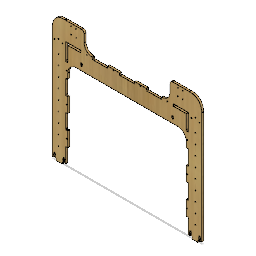
XZ1-plate-IIIS-rev1_8mm v1 (Autodesk Fusion 360 design; units mm, degrees)
Autodesk Fusion 360 part; units mm, degrees
sketch "Basic shape" plane through (0, 0, 0) normal (0, 0, 1) x (1, 0, 0)
  line L0 (-300, 500) -> (300, 500)
  line L1 (300, 500) -> (300, 0)
  line L2 (300, 0) -> (-300, 0)
  line L3 (-300, 0) -> (-300, 500)
  line L4 (-238, 0) -> (238, 0)
  line L5 (238, 0) -> (238, 355)
  line L6 (238, 355) -> (-238, 355)
  line L7 (-238, 355) -> (-238, 0)
  line L8 (300, 500) -> (247, 500)
  line L9 (247, 500) -> (247, 425)
  line L10 (247, 425) -> (300, 425)
  line L11 (300, 425) -> (300, 500)
  line L12 (-300, 500) -> (-247, 500)
  line L13 (-247, 500) -> (-247, 425)
  line L14 (-247, 425) -> (-300, 425)
  line L15 (-300, 425) -> (-300, 500)
  line L16 (247, 425) -> (172, 425)
  line L17 (172, 425) -> (172, 500)
  line L18 (172, 500) -> (247, 500)
  line L19 (247, 500) -> (247, 425)
  line L20 (-247, 425) -> (-172, 425)
  line L21 (-172, 425) -> (-172, 500)
  line L22 (-172, 500) -> (-247, 500)
  line L23 (-247, 500) -> (-247, 425)
  line L24 (-172, 500) -> (172, 500)
  line L25 (172, 500) -> (172, 425)
  line L26 (172, 425) -> (-172, 425)
  line L27 (-172, 425) -> (-172, 500)
  line L28 (-285.5, 0) -> (-260.5, 0)
  line L29 (-260.5, 0) -> (-260.5, -8)
  line L30 (-260.5, -8) -> (-285.5, -8)
  line L31 (-285.5, -8) -> (-285.5, 0)
  line L32 (260.5, 0) -> (285.5, 0)
  line L33 (285.5, 0) -> (285.5, -8)
  line L34 (285.5, -8) -> (260.5, -8)
  line L35 (260.5, -8) -> (260.5, 0)
  dimension "d1" = 500
  dimension "d2" = 600
  dimension "d3" = 53
  dimension "d4" = 53
  dimension "d6" = 62
  dimension "d7" = 75
  dimension "d8" = 75
  dimension "d9" = 75
  dimension "d11" = 25
  dimension "d12" = 8
  dimension "d14" = 14.5
  dimension "d15" = 14.5
  dimension "d16" = 8
  dimension "d17" = 25
  dimension "d102" = 70
  dimension "d111" = 18.5
  dimension "d112" = 23.5
  measures "d1" distance of origin
  measures "d3" distance of L1 L9
  measures "d4" distance of L13 L15
  measures "d6" distance of L1 L5
  measures "d7" distance of L21 L23
  measures "d8" distance of L17 L19
  measures "d9" distance of L24 L26
  measures "d12" distance of origin
  measures "d14" distance of origin L31
  measures "d15" distance of origin L33
  measures "d16" distance of origin
  measures "d102" distance of L6 L26
  measures "d111" distance of origin
extrude "Extrude1" add sketch "Basic shape" along normal blind 8 contours L0 L3 L12 L13 L14 L15 L23 | L0 L13 L20 L21 L22 L23 L27 | L1 L2 L3 L5 L6 L7 L10 L14 L16 L20 L26 L28 L32 | L0 L9 L16 L17 L18 L19 L25 | L2 L28 L29 L30 L31 | L0 L1 L8 L9 L10 L11 L19 | L2 L32 L33 L34 L35
fillet "Fillet1" radius 35 2 edges at (-238, 355, 4) (238, 355, 4)
fillet "Fillet2" radius 32.5 2 edges at (172, 425, 4) (-172, 425, 4)
fillet "Fillet3" radius 10 2 edges at (-172, 500, 4) (172, 500, 4)
sketch "Square+X projected" plane through (0, 0, 8) normal (0, 0, 1) x (1, 0, 0)
  line L0 (300, 500) -> (182, 500)
  arc A0 (182, 500) -> (172, 490) centre (182, 490) ccw
  line L1 (172, 490) -> (172, 457.5)
  arc A1 (139.5, 425) -> (172, 457.5) centre (139.5, 457.5) ccw
  line L2 (139.5, 425) -> (-139.5, 425)
  arc A2 (-172, 457.5) -> (-139.5, 425) centre (-139.5, 457.5) ccw
  line L3 (-172, 457.5) -> (-172, 490)
  arc A3 (-172, 490) -> (-182, 500) centre (-182, 490) ccw
  line L4 (-182, 500) -> (-247, 500)
  line L5 (-300, 0) -> (-285.5, 0)
  line L6 (-285.5, 0) -> (-285.5, -8)
  line L7 (-285.5, -8) -> (-260.5, -8)
  line L8 (-260.5, -8) -> (-260.5, 0)
  line L9 (-260.5, 0) -> (-238, 0)
  line L10 (-238, 0) -> (-238, 320)
  arc A4 (-203, 355) -> (-238, 320) centre (-203, 320) ccw
  line L11 (-203, 355) -> (203, 355)
  arc A5 (238, 320) -> (203, 355) centre (203, 320) ccw
  line L12 (238, 320) -> (238, 0)
  line L13 (238, 0) -> (260.5, 0)
  line L14 (260.5, 0) -> (260.5, -8)
  line L15 (260.5, -8) -> (285.5, -8)
  line L16 (285.5, -8) -> (285.5, 0)
  line L17 (285.5, 0) -> (300, 0)
  line L18 (300, 0) -> (300, 500)
  line L19 (-238, 0) -> (-246, 0) construction
  line L20 (-246, 0) -> (-246, 500) construction
  line L21 (-246, 500) -> (-238, 500) construction
  line L22 (-238, 500) -> (-238, 0) construction
  line L23 (-300, 425) -> (300, 425) construction
  line L24 (300, 425) -> (300, 417) construction
  line L25 (300, 417) -> (-300, 417) construction
  line L26 (-300, 417) -> (-300, 425) construction
  line L27 (-247, 500) -> (-300, 500)
  dimension "d27" = 8
  dimension "d34" = 8
  dimension "d107" = 75
sketch "Square+X joints" plane through (0, 0, 0) normal (0, 0, 1) x (1, 0, 0)
  line L0 (-238, 0) -> (-246, 0)
  line L1 (-246, 0) -> (-246, 60)
  line L2 (-246, 60) -> (-238, 60)
  line L3 (-238, 60) -> (-238, 0)
  line L4 (-246, 0) -> (-246, 500)
  line L5 (-238, 119) -> (-246, 119)
  line L6 (-246, 119) -> (-246, 179)
  line L7 (-246, 179) -> (-238, 179)
  line L8 (-238, 179) -> (-238, 119)
  line L9 (-238, 320) -> (-238, 0)
  line L10 (-238, 238) -> (-246, 238)
  line L11 (-246, 238) -> (-246, 298)
  line L12 (-246, 298) -> (-238, 298)
  line L13 (-238, 298) -> (-238, 238)
  line L14 (-246, 238) -> (-246, 179) construction
  line L15 (-246, 119) -> (-246, 60) construction
  line L16 (-238, 357) -> (-246, 357)
  line L17 (-246, 357) -> (-246, 417)
  line L18 (-246, 417) -> (-238, 417)
  line L19 (-238, 417) -> (-238, 357)
  line L20 (-246, 357) -> (-246, 298) construction
  line L21 (30, 425) -> (-30, 425)
  line L22 (-30, 425) -> (-30, 417)
  line L23 (-30, 417) -> (30, 417)
  line L24 (30, 417) -> (30, 425)
  line L25 (300, 417) -> (-300, 417)
  line L26 (-78, 425) -> (-138, 425)
  line L27 (-138, 425) -> (-138, 417)
  line L28 (-138, 417) -> (-78, 417)
  line L29 (-78, 417) -> (-78, 425)
  line L30 (-300, 425) -> (300, 425)
  line L31 (-186, 425) -> (-246, 425)
  line L32 (-30, 417) -> (-78, 417) construction
  line L33 (78, 425) -> (138, 425)
  line L34 (138, 425) -> (138, 417)
  line L35 (138, 417) -> (78, 417)
  line L36 (78, 417) -> (78, 425)
  line L37 (186, 425) -> (246, 425)
  line L38 (246, 425) -> (246, 417)
  line L39 (246, 417) -> (186, 417)
  line L40 (186, 417) -> (186, 425)
  line L41 (186, 417) -> (138, 417) construction
  line L42 (78, 417) -> (30, 417) construction
  line L43 (300, 417) -> (246, 417) construction
  line L44 (-138, 417) -> (-186, 417) construction
  line L45 (-186, 425) -> (-186, 417)
  line L46 (-246, 417) -> (-246, 425)
  line L47 (-246, 417) -> (-186, 417)
  line L48 (-246, 417) -> (-300, 417) construction
  dimension "d28" = 60
  dimension "d29" = 60
  dimension "d30" = 60
  dimension "d31" = 60
  dimension "d33" = 58.3333
  dimension "d35" = 60
  dimension "d36" = 60
  dimension "d37" = 60
  dimension "d44" = 31.6667
  dimension "d46" = 60
  dimension "d47" = 60
extrude "Extrude2" cut sketch "Square+X joints" along normal blind 8 contours L0 L1 L2 L3 L4 L9 | L4 L5 L6 L7 L8 L9 | L4 L9 L10 L11 L12 L13
extrude "Extrude3" cut sketch "Square+X joints" along normal through all contours L4 L16 L17 L18 L19 L25 L47 | L4 L18 L25 L30 L31 L45 L46 L47 | L25 L26 L27 L28 L29 L30 | L21 L22 L23 L24 L25 L30
mirror "Mirror1" about plane through (0, 0, 0) normal (1, 0, 0) of "Extrude2", "Extrude3"
sketch "Square+X joints holes" plane through (0, 0, 8) normal (0, 0, 1) x (1, 0, 0)
  line L0 (246, 60) -> (246, 0)
  line L1 (246, 0) -> (260.5, 0)
  line L2 (260.5, 0) -> (260.5, -8)
  line L3 (260.5, -8) -> (285.5, -8)
  line L4 (285.5, -8) -> (285.5, 0)
  line L5 (285.5, 0) -> (300, 0)
  line L6 (300, 0) -> (300, 500)
  line L7 (300, 500) -> (182, 500)
  arc A0 (182, 500) -> (172, 490) centre (182, 490) ccw
  line L8 (172, 490) -> (172, 457.5)
  arc A1 (139.5, 425) -> (172, 457.5) centre (139.5, 457.5) ccw
  line L9 (78, 425) -> (30, 425)
  arc A2 (-172, 457.5) -> (-139.5, 425) centre (-139.5, 457.5) ccw
  line L10 (-172, 457.5) -> (-172, 490)
  arc A3 (-172, 490) -> (-182, 500) centre (-182, 490) ccw
  line L11 (-182, 500) -> (-247, 500)
  line L12 (-300, 500) -> (-300, 0)
  line L13 (-300, 0) -> (-285.5, 0)
  line L14 (-285.5, 0) -> (-285.5, -8)
  line L15 (-285.5, -8) -> (-260.5, -8)
  line L16 (-260.5, -8) -> (-260.5, 0)
  line L17 (-260.5, 0) -> (-246, 0)
  line L18 (-246, 0) -> (-246, 60)
  line L19 (-246, 60) -> (-238, 60)
  line L20 (-238, 60) -> (-238, 119)
  line L21 (-238, 119) -> (-246, 119)
  line L22 (-246, 119) -> (-246, 179)
  line L23 (-246, 179) -> (-238, 179)
  line L24 (-238, 179) -> (-238, 238)
  line L25 (-238, 238) -> (-246, 238)
  line L26 (-246, 238) -> (-246, 298)
  line L27 (-246, 298) -> (-238, 298)
  arc A4 (-203, 355) -> (-238, 320) centre (-203, 320) ccw
  line L28 (-203, 355) -> (203, 355)
  arc A5 (238, 320) -> (203, 355) centre (203, 320) ccw
  line L29 (238, 298) -> (246, 298)
  line L30 (246, 298) -> (246, 238)
  line L31 (246, 238) -> (238, 238)
  line L32 (238, 320) -> (238, 298)
  line L33 (238, 179) -> (246, 179)
  line L34 (246, 179) -> (246, 119)
  line L35 (246, 119) -> (238, 119)
  line L36 (238, 119) -> (238, 60)
  line L37 (238, 60) -> (246, 60)
  circle A6 centre (-242, 89.5) radius 2
  circle A7 centre (-242, 208.5) radius 2
  circle A8 centre (-242, 327.338) radius 2
  circle A9 centre (-54, 421) radius 2
  circle A10 centre (-162, 421) radius 2
  line L38 (-30, 425) -> (-30, 417)
  circle A11 centre (-275, 421) radius 2
  line L39 (-30, 425) -> (-78, 425)
  line L40 (-246, 425) -> (-300, 500) construction
  line L41 (-138, 425) -> (-138, 417)
  line L42 (-138, 425) -> (-186, 425) construction
  line L43 (-247, 500) -> (-300, 500)
  line L44 (-238, 298) -> (-238, 320)
  line L45 (78, 417) -> (78, 425)
  line L46 (30, 425) -> (30, 417)
  line L47 (30, 417) -> (-30, 417)
  line L48 (-30, 417) -> (-30, 425)
  line L49 (-30, 425) -> (-78, 425)
  line L50 (-78, 425) -> (-78, 417)
  line L51 (-78, 417) -> (-138, 417)
  line L52 (-138, 417) -> (-138, 425)
  line L53 (-138, 425) -> (-139.5, 425)
  line L54 (238, 238) -> (238, 179)
  line L55 (139.5, 425) -> (138, 425)
  line L56 (138, 425) -> (138, 417)
  line L57 (138, 417) -> (78, 417)
  line L58 (238, 417) -> (186, 417)
  line L59 (186, 417) -> (186, 425)
  line L60 (186, 425) -> (246, 425)
  line L61 (246, 425) -> (246, 357)
  line L62 (246, 357) -> (238, 357)
  line L63 (238, 357) -> (238, 417)
  line L64 (-238, 357) -> (-246, 357)
  line L65 (-246, 357) -> (-246, 425)
  line L66 (-246, 425) -> (-186, 425)
  line L67 (-186, 425) -> (-186, 417)
  line L68 (-186, 417) -> (-238, 417)
  line L69 (-238, 417) -> (-238, 357)
  dimension "d49" = 29.1667
  dimension "d50" = 29.338
  dimension "d51" = 4
  dimension "d52" = 4
  dimension "d53" = 4
  dimension "d59" = 4
  dimension "d60" = 4
  dimension "d61" = 4
  dimension "d101" = 275
  measures "d51" diameter of A6
  measures "d52" diameter of A7
  measures "d53" diameter of A8
  measures "d59" diameter of A11
  measures "d60" diameter of A10
  measures "d61" diameter of A9
  measures "d101" distance of origin
extrude "Extrude4" cut sketch "Square+X joints holes" against normal through all contours A6 | A7 | A8 | A9 | A10 | A11
mirror "Mirror2" about plane through (0, 0, 0) normal (1, 0, 0) of "Extrude4"
sketch "Linear rail" plane through (0, 0, 8) normal (0, 0, 1) x (1, 0, 0)
  circle A0 centre (242, 89.5) radius 2
  circle A1 centre (162, 421) radius 2
  circle A2 centre (242, 208.5) radius 2
  circle A3 centre (275, 421) radius 2
  circle A4 centre (-54, 421) radius 2
  circle A5 centre (-242, 89.5) radius 2
  circle A6 centre (-162, 421) radius 2
  circle A7 centre (-242, 208.5) radius 2
  circle A8 centre (-275, 421) radius 2
  line L0 (246, 60) -> (246, 0)
  line L1 (246, 0) -> (260.5, 0)
  line L2 (260.5, 0) -> (260.5, -8)
  line L3 (260.5, -8) -> (285.5, -8)
  line L4 (285.5, -8) -> (285.5, 0)
  line L5 (285.5, 0) -> (300, 0)
  line L6 (300, 0) -> (300, 500)
  line L7 (300, 500) -> (182, 500)
  arc A9 (182, 500) -> (172, 490) centre (182, 490) ccw
  line L8 (172, 490) -> (172, 457.5)
  arc A10 (139.5, 425) -> (172, 457.5) centre (139.5, 457.5) ccw
  line L9 (78, 425) -> (30, 425)
  arc A11 (-172, 457.5) -> (-139.5, 425) centre (-139.5, 457.5) ccw
  line L10 (-172, 457.5) -> (-172, 490)
  arc A12 (-172, 490) -> (-182, 500) centre (-182, 490) ccw
  line L11 (-182, 500) -> (-247, 500)
  line L12 (-300, 500) -> (-300, 0)
  line L13 (-300, 0) -> (-285.5, 0)
  line L14 (-285.5, 0) -> (-285.5, -8)
  line L15 (-285.5, -8) -> (-260.5, -8)
  line L16 (-260.5, -8) -> (-260.5, 0)
  line L17 (-260.5, 0) -> (-246, 0)
  line L18 (-246, 0) -> (-246, 60)
  line L19 (-246, 60) -> (-238, 60)
  line L20 (-238, 60) -> (-238, 119)
  line L21 (-238, 119) -> (-246, 119)
  line L22 (-246, 119) -> (-246, 179)
  line L23 (-246, 179) -> (-238, 179)
  line L24 (-238, 179) -> (-238, 238)
  line L25 (-238, 238) -> (-246, 238)
  line L26 (-246, 238) -> (-246, 298)
  line L27 (-246, 298) -> (-238, 298)
  arc A13 (-203, 355) -> (-238, 320) centre (-203, 320) ccw
  line L28 (-203, 355) -> (203, 355)
  arc A14 (238, 320) -> (203, 355) centre (203, 320) ccw
  line L29 (238, 298) -> (246, 298)
  line L30 (246, 298) -> (246, 238)
  line L31 (246, 238) -> (238, 238)
  line L32 (238, 320) -> (238, 298)
  line L33 (238, 179) -> (246, 179)
  line L34 (246, 179) -> (246, 119)
  line L35 (246, 119) -> (238, 119)
  line L36 (238, 119) -> (238, 60)
  line L37 (238, 60) -> (246, 60)
  circle A15 centre (-275, 368.1667) radius 1.5
  line L38 (-247, 500) -> (-300, 500)
  circle A16 centre (54, 421) radius 2
  circle A17 centre (242, 327.338) radius 2
  circle A18 centre (-242, 327.338) radius 2
  line L39 (-238, 298) -> (-238, 320)
  line L40 (78, 417) -> (78, 425)
  line L41 (30, 425) -> (30, 417)
  line L42 (30, 417) -> (-30, 417)
  line L43 (-30, 417) -> (-30, 425)
  line L44 (-30, 425) -> (-78, 425)
  line L45 (-78, 425) -> (-78, 417)
  line L46 (-78, 417) -> (-138, 417)
  line L47 (-138, 417) -> (-138, 425)
  line L48 (-138, 425) -> (-139.5, 425)
  line L49 (238, 238) -> (238, 179)
  line L50 (139.5, 425) -> (138, 425)
  line L51 (138, 425) -> (138, 417)
  line L52 (138, 417) -> (78, 417)
  line L53 (238, 417) -> (186, 417)
  line L54 (186, 417) -> (186, 425)
  line L55 (186, 425) -> (246, 425)
  line L56 (246, 425) -> (246, 357)
  line L57 (246, 357) -> (238, 357)
  line L58 (238, 357) -> (238, 417)
  line L59 (-238, 357) -> (-246, 357)
  line L60 (-246, 357) -> (-246, 425)
  line L61 (-246, 425) -> (-186, 425)
  line L62 (-186, 425) -> (-186, 417)
  line L63 (-186, 417) -> (-238, 417)
  line L64 (-238, 417) -> (-238, 357)
  dimension "d63" = 275
  dimension "d64" = 3
  measures "d63" distance of origin
  measures "d64" diameter of A15
extrude "Extrude5" cut sketch "Linear rail" against normal through all contours A15
pattern_linear "R-Pattern1" count 9 spacing 40 along (0, -1, 0) of "Extrude5"
mirror "Mirror3" about plane through (0, 0, 0) normal (1, 0, 0) of "Extrude5", "R-Pattern1"
sketch "Motor fixation" plane through (0, 0, 8) normal (0, 0, 1) x (1, 0, 0)
  circle A0 centre (275, 368.1667) radius 1.5
  circle A1 centre (-275, 48.1667) radius 1.5
  circle A2 centre (-275, 88.1667) radius 1.5
  circle A3 centre (-275, 128.1667) radius 1.5
  circle A4 centre (-275, 168.1667) radius 1.5
  circle A5 centre (-275, 208.1667) radius 1.5
  circle A6 centre (-275, 248.1667) radius 1.5
  circle A7 centre (-275, 288.1667) radius 1.5
  circle A8 centre (-275, 328.1667) radius 1.5
  circle A9 centre (-275, 368.1667) radius 1.5
  circle A10 centre (242, 89.5) radius 2
  circle A11 centre (162, 421) radius 2
  circle A12 centre (242, 208.5) radius 2
  circle A13 centre (275, 421) radius 2
  circle A14 centre (-54, 421) radius 2
  circle A15 centre (-242, 89.5) radius 2
  circle A16 centre (-162, 421) radius 2
  circle A17 centre (-242, 208.5) radius 2
  circle A18 centre (-275, 421) radius 2
  line L0 (246, 60) -> (246, 0)
  line L1 (246, 0) -> (260.5, 0)
  line L2 (260.5, 0) -> (260.5, -8)
  line L3 (260.5, -8) -> (285.5, -8)
  line L4 (285.5, -8) -> (285.5, 0)
  line L5 (285.5, 0) -> (300, 0)
  line L6 (300, 0) -> (300, 500)
  line L7 (300, 500) -> (182, 500)
  arc A19 (182, 500) -> (172, 490) centre (182, 490) ccw
  line L8 (172, 490) -> (172, 457.5)
  arc A20 (139.5, 425) -> (172, 457.5) centre (139.5, 457.5) ccw
  line L9 (78, 425) -> (30, 425)
  arc A21 (-172, 457.5) -> (-139.5, 425) centre (-139.5, 457.5) ccw
  line L10 (-172, 457.5) -> (-172, 490)
  arc A22 (-172, 490) -> (-182, 500) centre (-182, 490) ccw
  line L11 (-182, 500) -> (-247, 500)
  line L12 (-300, 500) -> (-300, 0)
  line L13 (-300, 0) -> (-285.5, 0)
  line L14 (-285.5, 0) -> (-285.5, -8)
  line L15 (-285.5, -8) -> (-260.5, -8)
  line L16 (-260.5, -8) -> (-260.5, 0)
  line L17 (-260.5, 0) -> (-246, 0)
  line L18 (-246, 0) -> (-246, 60)
  line L19 (-246, 60) -> (-238, 60)
  line L20 (-238, 60) -> (-238, 119)
  line L21 (-238, 119) -> (-246, 119)
  line L22 (-246, 119) -> (-246, 179)
  line L23 (-246, 179) -> (-238, 179)
  line L24 (-238, 179) -> (-238, 238)
  line L25 (-238, 238) -> (-246, 238)
  line L26 (-246, 238) -> (-246, 298)
  line L27 (-246, 298) -> (-238, 298)
  arc A23 (-203, 355) -> (-238, 320) centre (-203, 320) ccw
  line L28 (-203, 355) -> (203, 355)
  arc A24 (238, 320) -> (203, 355) centre (203, 320) ccw
  line L29 (238, 298) -> (246, 298)
  line L30 (246, 298) -> (246, 238)
  line L31 (246, 238) -> (238, 238)
  line L32 (238, 320) -> (238, 298)
  line L33 (238, 179) -> (246, 179)
  line L34 (246, 179) -> (246, 119)
  line L35 (246, 119) -> (238, 119)
  line L36 (238, 119) -> (238, 60)
  line L37 (238, 60) -> (246, 60)
  line L38 (-229.5, 487.99) -> (-199.5, 487.99)
  arc A25 (-199.5, 487.99) -> (-199.5, 492.01) centre (-199.5, 490) ccw
  line L39 (-199.5, 492.01) -> (-229.5, 492.01)
  arc A26 (-229.5, 492.01) -> (-229.5, 487.99) centre (-229.5, 490) ccw
  line L40 (-229.5, 490) -> (-199.5, 490) construction
  line L41 (-229.5, 457.99) -> (-199.5, 457.99)
  arc A27 (-199.5, 457.99) -> (-199.5, 462.01) centre (-199.5, 460) ccw
  line L42 (-199.5, 462.01) -> (-229.5, 462.01)
  arc A28 (-229.5, 462.01) -> (-229.5, 457.99) centre (-229.5, 460) ccw
  line L43 (-229.5, 460) -> (-199.5, 460) construction
  line L44 (-214.5, 490) -> (-214.5, 460) construction
  circle A29 centre (275, 48.1667) radius 1.5
  circle A30 centre (275, 88.1667) radius 1.5
  circle A31 centre (275, 128.1667) radius 1.5
  circle A32 centre (275, 168.1667) radius 1.5
  circle A33 centre (275, 208.1667) radius 1.5
  circle A34 centre (275, 248.1667) radius 1.5
  circle A35 centre (275, 288.1667) radius 1.5
  circle A36 centre (275, 328.1667) radius 1.5
  line L45 (-247, 500) -> (-300, 500)
  circle A37 centre (54, 421) radius 2
  circle A38 centre (242, 327.338) radius 2
  circle A39 centre (-242, 327.338) radius 2
  line L46 (-238, 298) -> (-238, 320)
  line L47 (78, 417) -> (78, 425)
  line L48 (30, 425) -> (30, 417)
  line L49 (30, 417) -> (-30, 417)
  line L50 (-30, 417) -> (-30, 425)
  line L51 (-30, 425) -> (-78, 425)
  line L52 (-78, 425) -> (-78, 417)
  line L53 (-78, 417) -> (-138, 417)
  line L54 (-138, 417) -> (-138, 425)
  line L55 (-138, 425) -> (-139.5, 425)
  line L56 (238, 238) -> (238, 179)
  line L57 (139.5, 425) -> (138, 425)
  line L58 (138, 425) -> (138, 417)
  line L59 (138, 417) -> (78, 417)
  line L60 (238, 417) -> (186, 417)
  line L61 (186, 417) -> (186, 425)
  line L62 (186, 425) -> (246, 425)
  line L63 (246, 425) -> (246, 357)
  line L64 (246, 357) -> (238, 357)
  line L65 (238, 357) -> (238, 417)
  line L66 (-238, 357) -> (-246, 357)
  line L67 (-246, 357) -> (-246, 425)
  line L68 (-246, 425) -> (-186, 425)
  line L69 (-186, 425) -> (-186, 417)
  line L70 (-186, 417) -> (-238, 417)
  line L71 (-238, 417) -> (-238, 357)
  circle A40 centre (-204.5, 490) radius 2.01
  circle A41 centre (-224.5, 490) radius 2.01
  circle A42 centre (-204.5, 460) radius 2.01
  circle A43 centre (-224.5, 460) radius 2.01
  line L72 (-186, 380) -> (-186, 374)
  arc A44 (-186, 374) -> (-180, 374) centre (-183, 374) ccw
  line L73 (-180, 374) -> (-180, 380)
  arc A45 (-180, 380) -> (-186, 380) centre (-183, 380) ccw
  line L74 (-183, 380) -> (-183, 374) construction
  dimension "d73" = 30
  dimension "d74" = 30
  dimension "d75" = 30
  dimension "d76" = 2.01
  dimension "d77" = 2.01
  dimension "d512" = 10
  dimension "d513" = 20
  dimension "d514" = 10
  dimension "d515" = 20
  dimension "d517" = 10
  dimension "d519" = 183
  dimension "d520" = 380
  dimension "d521" = 6
  dimension "d522" = 3
  measures "d519" distance of origin
  measures "d520" distance of origin
  measures "d522" distance of L73
extrude "Extrude6" cut sketch "Motor fixation" against normal through all contours A41 | A40 | A43 | A42 | L72 A44 L73 A45
mirror "Mirror4" about plane through (0, 0, 0) normal (1, 0, 0) of "Extrude6"
sketch "T slots" plane through (0, 0, 8) normal (0, 0, 1) x (1, 0, 0)
  circle A0 centre (275, 368.1667) radius 1.5
  circle A1 centre (-275, 48.1667) radius 1.5
  circle A2 centre (-275, 88.1667) radius 1.5
  circle A3 centre (-275, 128.1667) radius 1.5
  circle A4 centre (-275, 168.1667) radius 1.5
  circle A5 centre (-275, 208.1667) radius 1.5
  circle A6 centre (-275, 248.1667) radius 1.5
  circle A7 centre (-275, 288.1667) radius 1.5
  circle A8 centre (-275, 328.1667) radius 1.5
  circle A9 centre (-275, 368.1667) radius 1.5
  circle A10 centre (242, 89.5) radius 2
  circle A11 centre (162, 421) radius 2
  circle A12 centre (242, 208.5) radius 2
  circle A13 centre (275, 421) radius 2
  circle A14 centre (-54, 421) radius 2
  circle A15 centre (-242, 89.5) radius 2
  circle A16 centre (-162, 421) radius 2
  circle A17 centre (-242, 208.5) radius 2
  circle A18 centre (-275, 421) radius 2
  line L0 (246, 60) -> (246, 0)
  line L1 (246, 0) -> (260.5, 0)
  line L2 (260.5, 0) -> (260.5, -8)
  line L3 (260.5, -8) -> (285.5, -8)
  line L4 (285.5, -8) -> (285.5, 0)
  line L5 (285.5, 0) -> (300, 0)
  line L6 (300, 0) -> (300, 500)
  line L7 (300, 500) -> (182, 500)
  arc A19 (182, 500) -> (172, 490) centre (182, 490) ccw
  line L8 (172, 490) -> (172, 457.5)
  arc A20 (139.5, 425) -> (172, 457.5) centre (139.5, 457.5) ccw
  line L9 (78, 425) -> (30, 425)
  arc A21 (-172, 457.5) -> (-139.5, 425) centre (-139.5, 457.5) ccw
  line L10 (-172, 457.5) -> (-172, 490)
  arc A22 (-172, 490) -> (-182, 500) centre (-182, 490) ccw
  line L11 (-182, 500) -> (-247, 500)
  line L12 (-300, 500) -> (-300, 0)
  line L13 (-300, 0) -> (-285.5, 0)
  line L14 (-285.5, 0) -> (-285.5, -8)
  line L15 (-285.5, -8) -> (-260.5, -8)
  line L16 (-260.5, -8) -> (-260.5, 0)
  line L17 (-260.5, 0) -> (-246, 0)
  line L18 (-246, 0) -> (-246, 60)
  line L19 (-246, 60) -> (-238, 60)
  line L20 (-238, 60) -> (-238, 119)
  line L21 (-238, 119) -> (-246, 119)
  line L22 (-246, 119) -> (-246, 179)
  line L23 (-246, 179) -> (-238, 179)
  line L24 (-238, 179) -> (-238, 238)
  line L25 (-238, 238) -> (-246, 238)
  line L26 (-246, 238) -> (-246, 298)
  line L27 (-246, 298) -> (-238, 298)
  arc A23 (-203, 355) -> (-238, 320) centre (-203, 320) ccw
  line L28 (-203, 355) -> (203, 355)
  arc A24 (238, 320) -> (203, 355) centre (203, 320) ccw
  line L29 (238, 298) -> (246, 298)
  line L30 (246, 298) -> (246, 238)
  line L31 (246, 238) -> (238, 238)
  line L32 (238, 320) -> (238, 298)
  line L33 (238, 179) -> (246, 179)
  line L34 (246, 179) -> (246, 119)
  line L35 (246, 119) -> (238, 119)
  line L36 (238, 119) -> (238, 60)
  line L37 (238, 60) -> (246, 60)
  line L38 (-293.51, 0) -> (-289.49, 0)
  line L39 (-289.49, 0) -> (-289.49, 17.5)
  line L40 (-289.49, 17.5) -> (-293.51, 17.5)
  line L41 (-293.51, 17.5) -> (-293.51, 0)
  line L42 (-294.98, 12.5) -> (-287.98, 12.5)
  line L43 (-287.98, 12.5) -> (-287.98, 5)
  line L44 (-287.98, 5) -> (-294.98, 5)
  line L45 (-294.98, 5) -> (-294.98, 12.5)
  circle A25 centre (275, 48.1667) radius 1.5
  circle A26 centre (275, 88.1667) radius 1.5
  circle A27 centre (275, 128.1667) radius 1.5
  circle A28 centre (275, 168.1667) radius 1.5
  circle A29 centre (275, 208.1667) radius 1.5
  circle A30 centre (275, 248.1667) radius 1.5
  circle A31 centre (275, 288.1667) radius 1.5
  circle A32 centre (275, 328.1667) radius 1.5
  line L46 (-247, 500) -> (-300, 500)
  circle A33 centre (54, 421) radius 2
  circle A34 centre (242, 327.338) radius 2
  circle A35 centre (-242, 327.338) radius 2
  line L47 (-238, 298) -> (-238, 320)
  line L48 (78, 417) -> (78, 425)
  line L49 (30, 425) -> (30, 417)
  line L50 (30, 417) -> (-30, 417)
  line L51 (-30, 417) -> (-30, 425)
  line L52 (-30, 425) -> (-78, 425)
  line L53 (-78, 425) -> (-78, 417)
  line L54 (-78, 417) -> (-138, 417)
  line L55 (-138, 417) -> (-138, 425)
  line L56 (-138, 425) -> (-139.5, 425)
  line L57 (139.5, 425) -> (138, 425)
  line L58 (138, 425) -> (138, 417)
  line L59 (138, 417) -> (78, 417)
  line L60 (238, 417) -> (186, 417)
  line L61 (186, 417) -> (186, 425)
  line L62 (186, 425) -> (246, 425)
  line L63 (246, 425) -> (246, 357)
  line L64 (246, 357) -> (238, 357)
  line L65 (238, 357) -> (238, 417)
  line L66 (-238, 357) -> (-246, 357)
  line L67 (-246, 357) -> (-246, 425)
  line L68 (-246, 425) -> (-186, 425)
  line L69 (-186, 425) -> (-186, 417)
  line L70 (-186, 417) -> (-238, 417)
  line L71 (-238, 417) -> (-238, 357)
  circle A36 centre (204.5, 490) radius 2.01
  circle A37 centre (224.5, 460) radius 2.01
  circle A38 centre (224.5, 490) radius 2.01
  circle A39 centre (204.5, 460) radius 2.01
  circle A40 centre (-204.5, 490) radius 2.01
  circle A41 centre (-224.5, 460) radius 2.01
  circle A42 centre (-224.5, 490) radius 2.01
  circle A43 centre (-204.5, 460) radius 2.01
  line L72 (186, 380) -> (186, 374)
  arc A44 (180, 374) -> (186, 374) centre (183, 374) ccw
  line L73 (180, 374) -> (180, 380)
  arc A45 (186, 380) -> (180, 380) centre (183, 380) ccw
  line L74 (-180, 380) -> (-180, 374)
  arc A46 (-186, 374) -> (-180, 374) centre (-183, 374) ccw
  line L75 (-186, 374) -> (-186, 380)
  arc A47 (-180, 380) -> (-186, 380) centre (-183, 380) ccw
  line L76 (238, 238) -> (238, 179)
  dimension "d82" = 4.02
  dimension "d84" = 7
  dimension "d85" = 7.5
  dimension "d86" = 5
  dimension "d87" = 17.5
  dimension "d103" = 1.51
  dimension "d511" = 6
  measures "d86" distance of origin L44
  measures "d87" distance of origin
  measures "d103" distance of origin
extrude "Extrude7" cut sketch "T slots" against normal through all contours L13 L38 L39 L41 L44 | L39 L41 L42 L44 | L39 L42 L43 L44 | L41 L42 L44 L45 | L39 L40 L41 L42
pattern_linear "R-Pattern2" count 2 spacing 37 along (1, 0, 0) of "Extrude7"
mirror "Mirror5" about plane through (0, 0, 0) normal (1, 0, 0) of "Extrude7", "R-Pattern2"
sketch "SK8" plane through (0, 0, 8) normal (0, 0, 1) x (1, 0, 0)
  circle A0 centre (275, 48.1667) radius 1.5
  circle A1 centre (275, 88.1667) radius 1.5
  circle A2 centre (275, 128.1667) radius 1.5
  circle A3 centre (275, 168.1667) radius 1.5
  circle A4 centre (275, 208.1667) radius 1.5
  circle A5 centre (275, 248.1667) radius 1.5
  circle A6 centre (275, 288.1667) radius 1.5
  circle A7 centre (275, 328.1667) radius 1.5
  circle A8 centre (275, 368.1667) radius 1.5
  circle A9 centre (-275, 48.1667) radius 1.5
  circle A10 centre (-275, 88.1667) radius 1.5
  circle A11 centre (-275, 128.1667) radius 1.5
  circle A12 centre (-275, 168.1667) radius 1.5
  circle A13 centre (-275, 208.1667) radius 1.5
  circle A14 centre (-275, 248.1667) radius 1.5
  circle A15 centre (-275, 288.1667) radius 1.5
  circle A16 centre (-275, 328.1667) radius 1.5
  circle A17 centre (-275, 368.1667) radius 1.5
  circle A18 centre (242, 89.5) radius 2
  circle A19 centre (162, 421) radius 2
  circle A20 centre (242, 208.5) radius 2
  circle A21 centre (275, 421) radius 2
  circle A22 centre (-54, 421) radius 2
  circle A23 centre (-242, 89.5) radius 2
  circle A24 centre (-162, 421) radius 2
  circle A25 centre (-242, 208.5) radius 2
  circle A26 centre (-275, 421) radius 2
  line L0 (252.49, 0) -> (252.49, 5)
  line L1 (252.49, 5) -> (250.98, 5)
  line L2 (250.98, 5) -> (250.98, 12.5)
  line L3 (250.98, 12.5) -> (252.49, 12.5)
  line L4 (252.49, 12.5) -> (252.49, 17.5)
  line L5 (252.49, 17.5) -> (256.51, 17.5)
  line L6 (256.51, 17.5) -> (256.51, 12.5)
  line L7 (256.51, 12.5) -> (257.98, 12.5)
  line L8 (257.98, 12.5) -> (257.98, 5)
  line L9 (257.98, 5) -> (256.51, 5)
  line L10 (256.51, 5) -> (256.51, 0)
  line L11 (260.5, 0) -> (260.5, -8)
  line L12 (260.5, -8) -> (285.5, -8)
  line L13 (285.5, -8) -> (285.5, 0)
  line L14 (285.5, 0) -> (289.49, 0)
  line L15 (289.49, 0) -> (289.49, 5)
  line L16 (289.49, 5) -> (287.98, 5)
  line L17 (287.98, 5) -> (287.98, 12.5)
  line L18 (287.98, 12.5) -> (289.49, 12.5)
  line L19 (289.49, 12.5) -> (289.49, 17.5)
  line L20 (289.49, 17.5) -> (293.51, 17.5)
  line L21 (293.51, 17.5) -> (293.51, 12.5)
  line L22 (293.51, 12.5) -> (294.98, 12.5)
  line L23 (294.98, 12.5) -> (294.98, 5)
  line L24 (294.98, 5) -> (293.51, 5)
  line L25 (293.51, 5) -> (293.51, 0)
  line L26 (293.51, 0) -> (300, 0)
  line L27 (300, 0) -> (300, 500)
  line L28 (300, 500) -> (182, 500)
  arc A27 (182, 500) -> (172, 490) centre (182, 490) ccw
  line L29 (172, 490) -> (172, 457.5)
  arc A28 (139.5, 425) -> (172, 457.5) centre (139.5, 457.5) ccw
  line L30 (139.5, 425) -> (138, 425)
  arc A29 (-172, 457.5) -> (-139.5, 425) centre (-139.5, 457.5) ccw
  line L31 (-172, 457.5) -> (-172, 490)
  arc A30 (-172, 490) -> (-182, 500) centre (-182, 490) ccw
  line L32 (-182, 500) -> (-247, 500)
  line L33 (-300, 500) -> (-300, 0)
  line L34 (-300, 0) -> (-293.51, 0)
  line L35 (-293.51, 0) -> (-293.51, 5)
  line L36 (-293.51, 5) -> (-294.98, 5)
  line L37 (-294.98, 5) -> (-294.98, 12.5)
  line L38 (-294.98, 12.5) -> (-293.51, 12.5)
  line L39 (-293.51, 12.5) -> (-293.51, 17.5)
  line L40 (-293.51, 17.5) -> (-289.49, 17.5)
  line L41 (-289.49, 17.5) -> (-289.49, 12.5)
  line L42 (-289.49, 12.5) -> (-287.98, 12.5)
  line L43 (-287.98, 12.5) -> (-287.98, 5)
  line L44 (-287.98, 5) -> (-289.49, 5)
  line L45 (-289.49, 5) -> (-289.49, 0)
  line L46 (-289.49, 0) -> (-285.5, 0)
  line L47 (-285.5, 0) -> (-285.5, -8)
  line L48 (-285.5, -8) -> (-260.5, -8)
  line L49 (-260.5, -8) -> (-260.5, 0)
  line L50 (-256.51, 0) -> (-256.51, 5)
  line L51 (-256.51, 5) -> (-257.98, 5)
  line L52 (-257.98, 5) -> (-257.98, 12.5)
  line L53 (-257.98, 12.5) -> (-256.51, 12.5)
  line L54 (-256.51, 12.5) -> (-256.51, 17.5)
  line L55 (-256.51, 17.5) -> (-252.49, 17.5)
  line L56 (-252.49, 17.5) -> (-252.49, 12.5)
  line L57 (-252.49, 12.5) -> (-250.98, 12.5)
  line L58 (-250.98, 12.5) -> (-250.98, 5)
  line L59 (-250.98, 5) -> (-252.49, 5)
  line L60 (-252.49, 5) -> (-252.49, 0)
  line L61 (-260.5, 0) -> (-256.51, 0)
  line L62 (-246, 0) -> (-246, 60)
  line L63 (-246, 60) -> (-238, 60)
  line L64 (-238, 60) -> (-238, 119)
  line L65 (-238, 119) -> (-246, 119)
  line L66 (-246, 119) -> (-246, 179)
  line L67 (-246, 179) -> (-238, 179)
  line L68 (-238, 179) -> (-238, 238)
  line L69 (-238, 238) -> (-246, 238)
  line L70 (-246, 238) -> (-246, 298)
  line L71 (-246, 298) -> (-238, 298)
  arc A31 (-203, 355) -> (-238, 320) centre (-203, 320) ccw
  line L72 (-203, 355) -> (203, 355)
  arc A32 (238, 320) -> (203, 355) centre (203, 320) ccw
  line L73 (238, 298) -> (246, 298)
  line L74 (246, 298) -> (246, 238)
  line L75 (246, 238) -> (238, 238)
  line L76 (238, 320) -> (238, 298)
  line L77 (238, 179) -> (246, 179)
  line L78 (246, 179) -> (246, 119)
  line L79 (246, 119) -> (238, 119)
  line L80 (238, 119) -> (238, 60)
  line L81 (238, 60) -> (246, 60)
  line L82 (246, 60) -> (246, 0)
  line L83 (256.51, 0) -> (260.5, 0)
  line L84 (-291, 412.5) -> (-259, 412.5) construction
  circle A33 centre (-291, 412.5) radius 2
  circle A34 centre (-259, 412.5) radius 2
  line L85 (-247, 500) -> (-300, 500)
  circle A35 centre (54, 421) radius 2
  circle A36 centre (242, 327.338) radius 2
  circle A37 centre (-242, 327.338) radius 2
  line L86 (-238, 298) -> (-238, 320)
  line L87 (138, 425) -> (138, 417)
  line L88 (138, 417) -> (78, 417)
  line L89 (78, 417) -> (78, 425)
  line L90 (78, 425) -> (30, 425)
  line L91 (30, 425) -> (30, 417)
  line L92 (30, 417) -> (-30, 417)
  line L93 (-30, 417) -> (-30, 425)
  line L94 (-30, 425) -> (-78, 425)
  line L95 (-78, 425) -> (-78, 417)
  line L96 (-78, 417) -> (-138, 417)
  line L97 (-138, 417) -> (-138, 425)
  line L98 (-138, 425) -> (-139.5, 425)
  line L99 (238, 417) -> (186, 417)
  line L100 (186, 417) -> (186, 425)
  line L101 (186, 425) -> (246, 425)
  line L102 (246, 425) -> (246, 357)
  line L103 (246, 357) -> (238, 357)
  line L104 (238, 357) -> (238, 417)
  line L105 (-238, 357) -> (-246, 357)
  line L106 (-246, 357) -> (-246, 425)
  line L107 (-246, 425) -> (-186, 425)
  line L108 (-186, 425) -> (-186, 417)
  line L109 (-186, 417) -> (-238, 417)
  line L110 (-238, 417) -> (-238, 357)
  circle A38 centre (204.5, 490) radius 2.01
  circle A39 centre (224.5, 460) radius 2.01
  circle A40 centre (224.5, 490) radius 2.01
  circle A41 centre (204.5, 460) radius 2.01
  circle A42 centre (-204.5, 490) radius 2.01
  circle A43 centre (-224.5, 460) radius 2.01
  circle A44 centre (-224.5, 490) radius 2.01
  circle A45 centre (-204.5, 460) radius 2.01
  line L111 (186, 380) -> (186, 374)
  arc A46 (180, 374) -> (186, 374) centre (183, 374) ccw
  line L112 (180, 374) -> (180, 380)
  arc A47 (186, 380) -> (180, 380) centre (183, 380) ccw
  line L113 (-180, 380) -> (-180, 374)
  arc A48 (-186, 374) -> (-180, 374) centre (-183, 374) ccw
  line L114 (-186, 374) -> (-186, 380)
  arc A49 (-180, 380) -> (-186, 380) centre (-183, 380) ccw
  line L115 (-252.49, 0) -> (-246, 0)
  line L116 (238, 238) -> (238, 179)
  line L117 (246, 0) -> (252.49, 0)
  dimension "d94" = 32
  dimension "d95" = 275
  dimension "d97" = 4
  dimension "d98" = 4
  measures "d95" distance of origin
  measures "d97" diameter of A33
  measures "d98" diameter of A34
extrude "Extrude8" cut sketch "SK8" against normal through all contours A33 | A34
mirror "Mirror6" about plane through (0, 0, 0) normal (1, 0, 0) of "Extrude8"
fillet "Fillet4" chord length 70 curvature continuous 2 edges at (300, 500, 4) (-300, 500, 4)
hole "Hole31" at (244.5858, 296.5858, 8) direction (0, 0, -1) diameter 4 end up to surface (8 mm away)
hole "Hole32" at (-244.5858, 358.4142, 8) direction (0, 0, -1) diameter 4 end up to surface (8 mm away)
hole "Hole33" at (244.5858, 239.4142, 8) direction (0, 0, -1) diameter 4 end up to surface (8 mm away)
hole "Hole34" at (-244.5858, 423.5858, 8) direction (0, 0, -1) diameter 4 end up to surface (8 mm away)
hole "Hole35" at (-28.5858, 418.4142, 8) direction (0, 0, -1) diameter 4 end up to surface (8 mm away)
hole "Hole36" at (244.5858, 58.5858, 8) direction (0, 0, -1) diameter 4 end up to surface (8 mm away)
hole "Hole37" at (-244.5858, 120.4142, 8) direction (0, 0, -1) diameter 4 end up to surface (8 mm away)
hole "Hole38" at (28.5858, 418.4142, 8) direction (0, 0, -1) diameter 4 end up to surface (8 mm away)
hole "Hole39" at (-244.5858, 296.5858, 8) direction (0, 0, -1) diameter 4 end up to surface (8 mm away)
hole "Hole40" at (239.4142, 358.4142, 8) direction (0, 0, -1) diameter 4 end up to surface (8 mm away)
hole "Hole41" at (-244.5858, 177.5858, 8) direction (0, 0, -1) diameter 4 end up to surface (8 mm away)
hole "Hole42" at (-187.4142, 423.5858, 8) direction (0, 0, -1) diameter 4 end up to surface (8 mm away)
hole "Hole43" at (244.5858, 423.5858, 8) direction (0, 0, -1) diameter 4 end up to surface (8 mm away)
hole "Hole44" at (-79.4142, 418.4142, 8) direction (0, 0, -1) diameter 4 end up to surface (8 mm away)
hole "Hole45" at (-286.9142, -1.4142, 8) direction (0, 0, -1) diameter 4 end up to surface (8 mm away)
hole "Hole46" at (-239.4142, 358.4142, 8) direction (0, 0, -1) diameter 4 end up to surface (8 mm away)
hole "Hole47" at (-187.4142, 418.4142, 8) direction (0, 0, -1) diameter 4 end up to surface (8 mm away)
hole "Hole48" at (-244.5858, 239.4142, 8) direction (0, 0, -1) diameter 4 end up to surface (8 mm away)
hole "Hole49" at (244.5858, 358.4142, 8) direction (0, 0, -1) diameter 4 end up to surface (8 mm away)
hole "Hole50" at (-259.0858, -1.4142, 8) direction (0, 0, -1) diameter 4 end up to surface (8 mm away)
hole "Hole51" at (79.4142, 418.4142, 8) direction (0, 0, -1) diameter 4 end up to surface (8 mm away)
hole "Hole52" at (187.4142, 423.5858, 8) direction (0, 0, -1) diameter 4 end up to surface (8 mm away)
hole "Hole53" at (-244.5858, 58.5858, 8) direction (0, 0, -1) diameter 4 end up to surface (8 mm away)
hole "Hole54" at (259.0858, -1.4142, 8) direction (0, 0, -1) diameter 4 end up to surface (8 mm away)
hole "Hole55" at (187.4142, 418.4142, 8) direction (0, 0, -1) diameter 4 end up to surface (8 mm away)
hole "Hole56" at (136.5858, 418.4142, 8) direction (0, 0, -1) diameter 4 end up to surface (8 mm away)
hole "Hole57" at (286.9142, -1.4142, 8) direction (0, 0, -1) diameter 4 end up to surface (8 mm away)
hole "Hole58" at (244.5858, 120.4142, 8) direction (0, 0, -1) diameter 4 end up to surface (8 mm away)
hole "Hole59" at (-136.5858, 418.4142, 8) direction (0, 0, -1) diameter 4 end up to surface (8 mm away)
hole "Hole60" at (244.5858, 177.5858, 8) direction (0, 0, -1) diameter 4 end up to surface (8 mm away)
equation "d12 = pannel_thickness"
equation "pannel_thickness = 8 mm"
equation "d16 = pannel_thickness"
equation "d18 = pannel_thickness"
equation "Square_joint_thickness = 60 mm"
equation "d27 = pannel_thickness"
equation "d28 = Square_joint_thickness"
equation "d29 = Square_joint_thickness"
equation "d30 = Square_joint_thickness"
equation "d31 = Square_joint_thickness"
equation "d34 = pannel_thickness"
equation "d35 = Square_joint_thickness"
equation "d36 = Square_joint_thickness"
equation "d37 = Square_joint_thickness"
equation "d38 = pannel_thickness"
equation "d46 = Square_joint_thickness"
equation "d47 = Square_joint_thickness"
equation "d50 = ( ( 58.676 / 2 ) * 1 mm )"
equation "d51 = tslot_diameter"
equation "d52 = tslot_diameter"
equation "d53 = tslot_diameter"
equation "d59 = tslot_diameter"
equation "d60 = tslot_diameter"
equation "d61 = tslot_diameter"
equation "d82 = tslot_diameter + 0.02 mm"
equation "d103 = ( 7 mm - tslot_diameter ) / 2 + 0.01 mm"
equation "tslot_diameter = 4 mm"
equation "dbToolDia = 4 mm"
equation "dbOffset = 0 mm" comment "Do NOT change formula"
equation "dbRadius = ( dbToolDia + dbOffset ) / 2" comment "Do NOT change formula"
equation "dbMinPercent = 10"
equation "dbHoleOffset = dbRadius / sqrt(2)" comment "Do NOT change formula"
equation "d524 = dbRadius * 2"
equation "d526 = dbHoleOffset"
equation "d527 = dbHoleOffset"
equation "d529 = dbRadius * 2"
equation "d531 = dbHoleOffset"
equation "d532 = dbHoleOffset"
equation "d534 = dbRadius * 2"
equation "d536 = dbHoleOffset"
equation "d537 = dbHoleOffset"
equation "d539 = dbRadius * 2"
equation "d541 = dbHoleOffset"
equation "d542 = dbHoleOffset"
equation "d544 = dbRadius * 2"
equation "d546 = dbHoleOffset"
equation "d547 = dbHoleOffset"
equation "d549 = dbRadius * 2"
equation "d551 = dbHoleOffset"
equation "d552 = dbHoleOffset"
equation "d554 = dbRadius * 2"
equation "d556 = dbHoleOffset"
equation "d557 = dbHoleOffset"
equation "d559 = dbRadius * 2"
equation "d561 = dbHoleOffset"
equation "d562 = dbHoleOffset"
equation "d564 = dbRadius * 2"
equation "d566 = dbHoleOffset"
equation "d567 = dbHoleOffset"
equation "d569 = dbRadius * 2"
equation "d571 = dbHoleOffset"
equation "d572 = dbHoleOffset"
equation "d574 = dbRadius * 2"
equation "d576 = dbHoleOffset"
equation "d577 = dbHoleOffset"
equation "d579 = dbRadius * 2"
equation "d581 = dbHoleOffset"
equation "d582 = dbHoleOffset"
equation "d584 = dbRadius * 2"
equation "d586 = dbHoleOffset"
equation "d587 = dbHoleOffset"
equation "d589 = dbRadius * 2"
equation "d591 = dbHoleOffset"
equation "d592 = dbHoleOffset"
equation "d594 = dbRadius * 2"
equation "d596 = dbHoleOffset"
equation "d597 = dbHoleOffset"
equation "d599 = dbRadius * 2"
equation "d601 = dbHoleOffset"
equation "d602 = dbHoleOffset"
equation "d604 = dbRadius * 2"
equation "d606 = dbHoleOffset"
equation "d607 = dbHoleOffset"
equation "d609 = dbRadius * 2"
equation "d611 = dbHoleOffset"
equation "d612 = dbHoleOffset"
equation "d614 = dbRadius * 2"
equation "d616 = dbHoleOffset"
equation "d617 = dbHoleOffset"
equation "d619 = dbRadius * 2"
equation "d621 = dbHoleOffset"
equation "d622 = dbHoleOffset"
equation "d624 = dbRadius * 2"
equation "d626 = dbHoleOffset"
equation "d627 = dbHoleOffset"
equation "d629 = dbRadius * 2"
equation "d631 = dbHoleOffset"
equation "d632 = dbHoleOffset"
equation "d634 = dbRadius * 2"
equation "d636 = dbHoleOffset"
equation "d637 = dbHoleOffset"
equation "d639 = dbRadius * 2"
equation "d641 = dbHoleOffset"
equation "d642 = dbHoleOffset"
equation "d644 = dbRadius * 2"
equation "d646 = dbHoleOffset"
equation "d647 = dbHoleOffset"
equation "d649 = dbRadius * 2"
equation "d651 = dbHoleOffset"
equation "d652 = dbHoleOffset"
equation "d654 = dbRadius * 2"
equation "d656 = dbHoleOffset"
equation "d657 = dbHoleOffset"
equation "d659 = dbRadius * 2"
equation "d661 = dbHoleOffset"
equation "d662 = dbHoleOffset"
equation "d664 = dbRadius * 2"
equation "d666 = dbHoleOffset"
equation "d667 = dbHoleOffset"
equation "d669 = dbRadius * 2"
equation "d671 = dbHoleOffset"
equation "d672 = dbHoleOffset"
